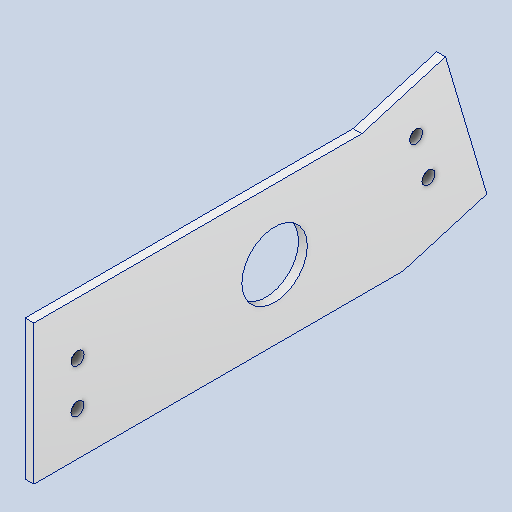
# Autodesk Inventor part: dribl-v1-Plate-6
Saved by Autodesk Inventor 2025.2 (Build 292293000, 293)
## iProperties
Created: 2025-01-07
Part Number: dribl-v1-Plate-6
Material: アルミニウム 6061
Document SubType Name: Modeling
Designer: haruy
Density: 2.7 g/cm^3
Appearance: アルミニウム - フラット
Author: haruy
Autodesk Inventor part; units mm, degrees
ref_plane "YZ Plane" through (0, 0, 0) normal (1, 0, 0) x (0, 1, 0)
ref_plane "XZ Plane" through (0, 0, 0) normal (0, 1, 0) x (-1, 0, 0)
ref_plane "XY Plane" through (0, 0, 0) normal (0, 0, 1) x (1, 0, 0)
derived "dribl-v1-ASP-Base.ipt"
sketch "スケッチ3" plane through (420, -432.3334, -303) normal (1, 0, 0) x (0, 0, -1)
  line L0 (20, 0) -> (20, 1308) projected
  line L1 (20, 102) -> (425, 102) projected
  line L2 (425, 102) -> (425, 122) projected
  line L3 (425, 122) -> (20, 122) projected
  line L4 (20, 122) -> (20, 102) projected
  circle A0 centre (55.18, 149) radius 21 projected
  circle A1 centre (55.18, 191) radius 16 projected
  circle A2 centre (55.18, 191) radius 13.68 projected
  line L5 (0, 0) -> (20, 0) projected
  line L6 (0, 0) -> (20, 0) projected
  line L7 (0, 0) -> (484, 0) projected
  line L8 (484, 0) -> (484, -20) projected
  line L9 (484, -20) -> (0, -20) projected
  line L10 (0, -20) -> (0, 0) projected
  line L11 (75.18, 1308) -> (94.3557, 1313.6826) projected
  line L12 (94.3557, 1313.6826) -> (480.203, 11.6512) projected
  line L13 (480.203, 11.6512) -> (461.0273, 5.9686) projected
  line L14 (461.0273, 5.9686) -> (75.18, 1308) projected
  line L15 (0, 1308) -> (0, 0) projected
  line L16 (0, 207) -> (55.18, 207) projected
  line L17 (76.18, 149) -> (76.18, 102) projected
  line L18 (76.18, 149) -> (76.18, 207) projected
  line L19 (76.18, 207) -> (55.18, 207) projected
  circle A3 centre (10, 195) radius 1.5 projected
  circle A4 centre (10, 185) radius 1.5 projected
  line L20 (55.18, 175) -> (0, 175) projected
  circle A5 centre (30, 112) radius 1.5 projected
  circle A6 centre (50, 112) radius 1.5 projected
  line L21 (20, 102) -> (0, 102) projected
  circle A7 centre (10, 112) radius 1.5 projected
  circle A8 centre (10, 132) radius 1.5 projected
  circle A9 centre (55.18, 1292) radius 16 projected
  line L22 (20, 1308) -> (0, 1308) projected
  line L23 (0, 1308) -> (55.18, 1308) projected
  line L24 (55.18, 1276) -> (0, 1276) projected
  line L25 (55.18, 1308) -> (75.18, 1308) projected
  circle A10 centre (55.18, 1292) radius 7.5 projected
  line L26 (55.18, 1276) -> (84.663, 1276) projected
  circle A11 centre (10, 1296) radius 1.5 projected
  circle A12 centre (10, 1286) radius 1.5 projected
  circle A13 centre (87.6092, 1301.2534) radius 1.5 projected
  circle A14 centre (90.4504, 1291.6656) radius 1.5 projected
  line L27 (84.663, 1276) -> (103.8387, 1281.6826) projected
  point P0 (-303, 432.3334)
  point P1 (55.18, 1308)
  constraints: 1 horizontal alignment
extrude "押し出し1" add sketch "スケッチ3" against normal blind 2 contours L24 L15 L22 L0 | L0 L23 A9 L24 | A9 | A9 L25 L14 L26 | L14 L11 L12 L27
